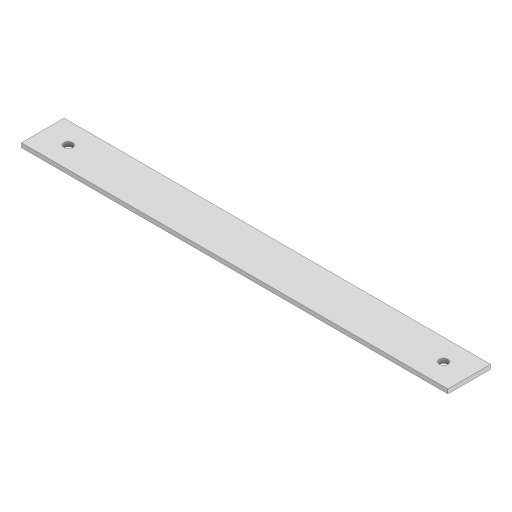
# Autodesk Inventor part: PLETINA PARA CARA INCLINADA
Saved by Autodesk Inventor 2024 (Build 280153000, 153)
## iProperties
Created: 2024-06-13
Part Number: PLETINA PARA CARA INCLINADA
Material: Generic
Document SubType Name: Modeling
Designer: Jhuliams
Density: 1 g/cm^3
Appearance: Default
Author: Jhuliams
Autodesk Inventor part; units mm, degrees
ref_plane "YZ Plane" through (0, 0, 0) normal (1, 0, 0) x (0, 1, 0)
ref_plane "XZ Plane" through (0, 0, 0) normal (0, 1, 0) x (-1, 0, 0)
ref_plane "XY Plane" through (0, 0, 0) normal (0, 0, 1) x (1, 0, 0)
sketch "Sketch1" plane through (0, 0, 0) normal (1, 0, 0) x (0, 1, 0)
  line L0 (1.25, 12.5) -> (-1.25, 12.5)
  line L1 (-1.25, 12.5) -> (-1.25, -12.5)
  line L2 (-1.25, -12.5) -> (1.25, -12.5)
  line L3 (1.25, -12.5) -> (1.25, 12.5)
  line L4 (1.25, 12.5) -> (-1.25, -12.5) construction
  line L5 (-1.25, 12.5) -> (1.25, -12.5) construction
  point P0 (0, 0)
  dimension "d0" = 2.5
  dimension "d1" = 25
  constraints: 12 end point, 2 midpoint, 2 parallel, 1 horizontal, 1 perpendicular
  measures "d0" distance of L2.end L1.end
  measures "d1" distance of L1.end L0.end
extrude "Extrusion1" add sketch "Sketch1" along normal mid plane 250
sketch "Sketch2" plane through (-125, 1.25, 12.5) normal (0, 1, 0) x (1, 0, 0)
  line L0 (0, 0) -> (0, 25) projected
  line L1 (0, 12.5) -> (15, 12.5)
  line L2 (15, 12.5) -> (235, 12.5)
  circle A0 centre (15, 12.5) radius 2.5
  circle A1 centre (235, 12.5) radius 2.5
  point P0 (125, 12.5)
  dimension "d4" = 15
  dimension "d5" = 220
  dimension "d6" = 5
  dimension "d7" = 5
  constraints: 4 end point, 2 centre point, 2 coincident, 2 point on line, 1 horizontal, 1 midpoint
  measures "d4" distance of L1.start L1.end
  measures "d5" distance of L1.end L2.end
  measures "d6" diameter of A0
  measures "d7" diameter of A1
extrude "Extrusion2" cut sketch "Sketch2" against normal blind 250
body "Solid1"
